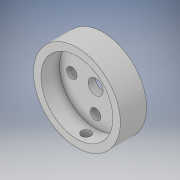
# Autodesk Inventor part: Input
Saved by Autodesk Inventor 2019.1 (Build 231200000, 200)
## iProperties
Created: 2019-01-08
Part Number: Input
Material: Generisch
Document SubType Name: Modeling
Designer: JochenAlt
Density: 1 g/cm^3
Appearance: Vorgabe
Author: JochenAlt
Autodesk Inventor part; units mm, degrees
ref_plane "YZ Plane" through (0, 0, 0) normal (1, 0, 0) x (0, 1, 0)
ref_plane "XZ Plane" through (0, 0, 0) normal (0, 1, 0) x (-1, 0, 0)
ref_plane "XY Plane" through (0, 0, 0) normal (0, 0, 1) x (1, 0, 0)
sketch "Skizze1" plane through (0, 0, 0) normal (0, 0, 1) x (1, 0, 0)
  circle A0 centre (0, 0) radius 2
  circle A1 centre (0, 0) radius 9.6
  circle A2 centre (0, 0) radius 6.35 construction
  circle A3 centre (6.35, 0) radius 1.4
  circle A4 centre (-6.35, 0) radius 1.4
  circle A5 centre (0, 6.35) radius 1.4
  circle A6 centre (0, -6.35) radius 1.4
  circle A7 centre (0, 0) radius 11.6
  circle A8 centre (0, 0) radius 4.3516
  line L0 (0, 16.24) -> (0, -16.24) construction
  line L1 (-16.24, 0) -> (16.24, 0) construction
  dimension "d0" = 19.2
  dimension "d1" = 12.7
  dimension "d2" = 2.8
  dimension "d3" = 4
  dimension "d4" = 2
  dimension "d5" = 8.7031
  constraints: 9 centre point, 8 coincident, 4 point on circle, 3 equal radius, 6 other
  measures "d0" diameter of A1
  measures "d1" diameter of A2
  measures "d2" diameter of A3
  measures "d3" diameter of A0
  measures "d4" radial gap between concentric circles of A1 A7
  measures "d5" diameter of A8
extrude "Extrusion1" add sketch "Skizze1" along normal blind 2 contours A1 | A7 | A8
extrude "Extrusion2" add sketch "Skizze1" along normal blind 5 from surface at 2 contours A7
sketch "Skizze2" plane through (0, 0, 0) normal (0, 1, 0) x (-1, 0, 0)
  circle A0 centre (0, 4.5) radius 1.25
  line L0 (9.6, 7) -> (-9.6, 7) projected
  point P0 (0, 0)
  dimension "d10" = 2.5
  dimension "d11" = 2.5
  constraints: 1 centre point
  measures "d10" diameter of A0
  measures "d11" distance from line of L0 A0.centre
extrude "Extrusion3" cut sketch "Skizze2" against normal through all
